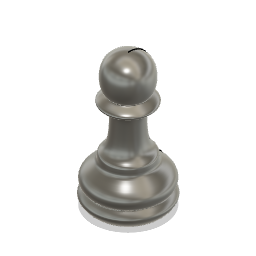
piyon (Autodesk Fusion 360 design; units mm, degrees)
Autodesk Fusion 360 part; units mm, degrees
sketch "Eskiz1" plane through (0, 0, 0) normal (1, 0, 0) x (0, 0, -1)
  spline S0 degree 5 poles (-0.001943, 29.955536) (0.53702, 29.934354) (1.576844, 29.850677) (3.02226, 29.601238) (4.71802, 29.031079) (6.43929, 27.982849) (7.755383, 26.673353) (8.671264, 25.177979) (9.222147, 23.54244) (9.462576, 21.793899) (9.529321, 19.847438) (9.391075, 17.847091) (8.956378, 16.058465) (8.220936, 14.727604) (7.349072, 13.970718) (6.890883, 13.619964) (7.72108, 13.144244) (9.270699, 12.436312) (10.631768, 11.537275) (10.897732, 10.63822) (9.94727, 9.925879) (8.379534, 9.33073) (6.940027, 8.672964) (6.274505, 7.725547) (6.137127, 6.279625) (6.159877, 4.310412) (6.257579, 1.951507) (6.401312, -0.574044) (6.648786, -3.004875) (7.065887, -5.098799) (7.692722, -6.690285) (8.496115, -7.741673) (9.312982, -8.41411) (9.937, -8.971389) (10.228366, -9.6584) (10.222813, -10.581822) (10.219179, -11.609183) (10.524579, -12.549279) (11.267438, -13.284313) (12.080255, -13.981948) (12.975568, -14.729301) (14.018323, -15.606311) (15.219428, -16.670967) (16.255196, -18.044099) (16.454373, -19.803048) (15.904981, -21.379825) (15.021112, -22.346416) (14.358806, -22.454071) (14.685283, -22.81832) (15.750122, -23.810713) (16.690838, -24.976603) (16.758628, -25.920253) (16.162715, -27.086046) (15.182399, -28.344591) (14.08355, -29.382898) (13.056821, -29.880556) (12.078169, -29.903784) (10.953809, -29.843456) (9.583568, -29.806806) (7.873524, -29.852749) (5.766463, -29.943995) (3.731699, -30.002959) (2.000704, -30.008153) (0.754872, -29.989854) (0.109001, -29.975257) knots 0 0 0 0 0 0 0.01666667 0.03333333 0.05 0.06666667 0.08333333 0.1 0.11666667 0.13333333 0.15 0.16666667 0.18333333 0.2 0.21666667 0.23333333 0.25 0.26666667 0.28333333 0.3 0.31666667 0.33333333 0.35 0.36666667 0.38333333 0.4 0.41666667 0.43333333 0.45 0.46666667 0.48333333 0.5 0.51666667 0.53333333 0.55 0.56666667 0.58333333 0.6 0.61666667 0.63333333 0.65 0.66666667 0.68333333 0.7 0.71666667 0.73333333 0.75 0.76666667 0.78333333 0.8 0.81666667 0.83333333 0.85 0.86666667 0.88333333 0.9 0.91666667 0.93333333 0.95 0.96666667 0.98333333 1 1 1 1 1 1
  line L0 (8.496587, 29.029558) -> (10.208824, 15.687386)
  line L1 (8.980407, 15.963471) -> (5.574509, 11.804789)
  line L2 (8.572913, 15.539688) -> (12.573268, 6.914504)
  line L3 (8.476183, 12.10685) -> (4.500794, 3.507028)
  line L4 (7.015836, -8.338009) -> (14.804353, -17.424613)
  line L5 (16.183168, -20.990334) -> (13.101017, -23.919061)
  line L6 (16.061875, -19.777395) -> (17.1977, -31.13565)
  line L7 (17.076004, -28.863999) -> (8.800704, -30.729998)
  line L8 (11.96479, -30.243215) -> (-11.746788, -29.707298)
  line L9 (10.463877, -10.366269) -> (20.524046, -23.915045)
  line L10 (-9.291373, 30.320623) -> (9.287487, 29.590449)
  line L11 (-0.001943, 29.955536) -> (0.109001, -29.975257)
  point P0 (9.352706, 22.358472)
  point P1 (7.277458, 13.88413)
  point P2 (10.573091, 11.227096)
  point P3 (6.488488, 7.806939)
  point P4 (7.848067, -6.758058)
  point P5 (10.139356, -9.636096)
  point P6 (10.910095, -12.881311)
  point P7 (15.493962, -17.140657)
  point P8 (14.642093, -22.454698)
  point P9 (16.629787, -25.456522)
  point P10 (12.938354, -29.796998)
revolve "Döndür1" add sketch "Eskiz1" angle 360 about axis through (0, 29.955536, 0.001943) along (0, -0.999998, -0.001851) contours S0 L1 L5 L11 | S0 L1 | S0 L5 picked at (2.105237, 2.191423) picked at (7.833524, 14.533935) picked at (15.230928, -21.949485)
